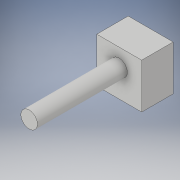
# Autodesk Inventor part: galvo
Saved by Autodesk Inventor 2019 (Build 230136000, 136)
## iProperties
Created: 2019-03-06
Part Number: galvo
Material: Generic
Document SubType Name: Modeling
Designer: Saumya
Density: 1 g/cm^3
Appearance: Default
Author: Saumya
Autodesk Inventor part; units mm, degrees
ref_plane "YZ Plane" through (0, 0, 0) normal (1, 0, 0) x (0, 1, 0)
ref_plane "XZ Plane" through (0, 0, 0) normal (0, 1, 0) x (-1, 0, 0)
ref_plane "XY Plane" through (0, 0, 0) normal (0, 0, 1) x (1, 0, 0)
sketch "Sketch3" plane through (0, 0, 0) normal (0, 0, 1) x (1, 0, 0)
  line L0 (51.7998, 73.9071) -> (77.1998, 73.9071)
  line L1 (77.1998, 73.9071) -> (77.1998, 48.5071)
  line L2 (77.1998, 48.5071) -> (51.7998, 48.5071)
  line L3 (51.7998, 48.5071) -> (51.7998, 73.9071)
  point P0 (0, 0)
  dimension "d2" = 25.4
  dimension "d3" = 25.4
  constraints: 8 end point, 2 parallel, 1 horizontal, 1 perpendicular
  measures "d2" distance of L0.end L1.end
  measures "d3" distance of L0.start L0.end
extrude "Extrusion2" add sketch "Sketch3" along normal blind 17.78
sketch "Sketch4" plane through (0, 0, 17.78) normal (0, 0, 1) x (1, 0, 0)
  circle A0 centre (64.4141, 63.8936) radius 4.6626
  point P0 (0, 0)
  constraints: 1 centre point
extrude "Extrusion3" add sketch "Sketch4" along normal blind 50.8
body "Solid2"
